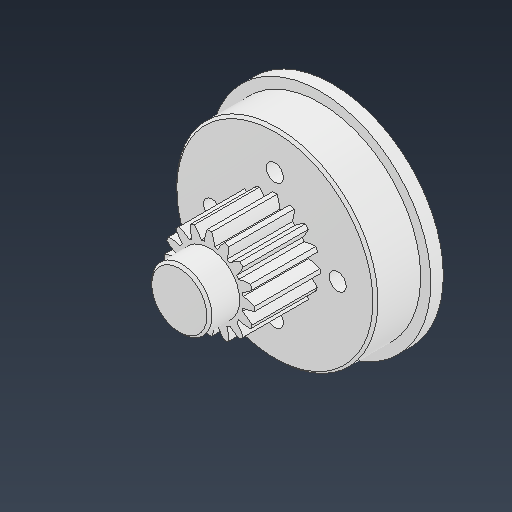
# Autodesk Inventor part: s-assy-sun_gear
Saved by Autodesk Inventor 2021 (Build 250183000, 183)
## iProperties
Created: 2021-07-12
Part Number: s-assy-sun_gear
Material: ABS プラスチック
Document SubType Name: Modeling
Designer: yuta0
Density: 1.06 g/cm^3
Appearance: 滑らか - 白
購入先: 印刷
在庫数: 0.0
Author: yuta0
Autodesk Inventor part; units mm, degrees
ref_plane "YZ Plane" through (0, 0, 0) normal (1, 0, 0) x (0, 1, 0)
ref_plane "XZ Plane" through (0, 0, 0) normal (0, 1, 0) x (-1, 0, 0)
ref_plane "XY Plane" through (0, 0, 0) normal (0, 0, 1) x (1, 0, 0)
sketch "スケッチ1" plane through (0, 0, 0) normal (1, 0, 0) x (0, 1, 0)
  line L0 (22, 0) -> (22, 2.5)
  line L1 (22, 2.5) -> (20, 2.5)
  line L2 (20, 2.5) -> (20, 11.5)
  line L3 (20, 11.5) -> (0, 11.5)
  line L4 (0, 11.5) -> (0, 0)
  line L5 (0, 0) -> (22, 0)
  dimension "d0" = 20
  dimension "d1" = 9
  dimension "d2" = 2.5
  dimension "d3" = 2
  constraints: 12 end point, 5 perpendicular, 1 vertical
  measures "d0" distance of L2.end L3.end
  measures "d1" distance of L1.end L2.end
  measures "d2" distance of L0.start L0.end
  measures "d3" distance of L0.end L1.end
revolve "回転1" add sketch "スケッチ1" angle 360 about axis through (0, 0, 11.5) along (0, 0, -1)
sketch "スケッチ2" plane through (0, 0, 11.5) normal (0, 0, 1) x (1, 0, 0)
  arc A0 (-3.8476, 8.135) -> (-3.4702, 5.7897) centre (3.494, 8.1133) ccw
  arc A1 (-3.4702, 5.7897) -> (-4.021, 5.4217) centre (0, 0) ccw
  arc A2 (-4.021, 5.4217) -> (-6.0434, 6.6678) centre (-8.8328, -0.1232) ccw
  arc A3 (-6.0434, 6.6678) -> (-6.6678, 6.0434) centre (0, 0) ccw
  arc A4 (-6.6678, 6.0434) -> (-5.4217, 4.021) centre (0.1232, 8.8328) ccw
  arc A5 (-5.4217, 4.021) -> (-5.7897, 3.4702) centre (0, 0) ccw
  arc A6 (-5.7897, 3.4702) -> (-8.135, 3.8476) centre (-8.1133, -3.494) ccw
  arc A7 (-8.135, 3.8476) -> (-8.473, 3.0317) centre (0, 0) ccw
  arc A8 (-8.473, 3.0317) -> (-6.5477, 1.6401) centre (-3.2664, 8.2076) ccw
  arc A9 (-6.5477, 1.6401) -> (-6.6769, 0.9904) centre (0, 0) ccw
  arc A10 (-6.6769, 0.9904) -> (-8.9882, 0.4416) centre (-6.1586, -6.3328) ccw
  arc A11 (-8.9882, 0.4416) -> (-8.9882, -0.4416) centre (0, 0) ccw
  arc A12 (-8.9882, -0.4416) -> (-6.6769, -0.9904) centre (-6.1586, 6.3328) ccw
  arc A13 (-6.6769, -0.9904) -> (-6.5477, -1.6401) centre (0, 0) ccw
  arc A14 (-6.5477, -1.6401) -> (-8.473, -3.0317) centre (-3.2664, -8.2076) ccw
  arc A15 (-8.473, -3.0317) -> (-8.135, -3.8476) centre (0, 0) ccw
  arc A16 (-8.135, -3.8476) -> (-5.7897, -3.4702) centre (-8.1133, 3.494) ccw
  arc A17 (-5.7897, -3.4702) -> (-5.4217, -4.021) centre (0, 0) ccw
  arc A18 (-5.4217, -4.021) -> (-6.6678, -6.0434) centre (0.1232, -8.8328) ccw
  arc A19 (-6.6678, -6.0434) -> (-6.0434, -6.6678) centre (0, 0) ccw
  arc A20 (-6.0434, -6.6678) -> (-4.021, -5.4217) centre (-8.8328, 0.1232) ccw
  arc A21 (-4.021, -5.4217) -> (-3.4702, -5.7897) centre (0, 0) ccw
  arc A22 (-3.4702, -5.7897) -> (-3.8476, -8.135) centre (3.494, -8.1133) ccw
  arc A23 (-3.8476, -8.135) -> (-3.0317, -8.473) centre (0, 0) ccw
  arc A24 (-3.0317, -8.473) -> (-1.6401, -6.5477) centre (-8.2076, -3.2664) ccw
  arc A25 (-1.6401, -6.5477) -> (-0.9904, -6.6769) centre (0, 0) ccw
  arc A26 (-0.9904, -6.6769) -> (-0.4416, -8.9882) centre (6.3328, -6.1586) ccw
  arc A27 (-0.4416, -8.9882) -> (0.4416, -8.9882) centre (0, 0) ccw
  arc A28 (0.4416, -8.9882) -> (0.9904, -6.6769) centre (-6.3328, -6.1586) ccw
  arc A29 (0.9904, -6.6769) -> (1.6401, -6.5477) centre (0, 0) ccw
  arc A30 (1.6401, -6.5477) -> (3.0317, -8.473) centre (8.2076, -3.2664) ccw
  arc A31 (3.0317, -8.473) -> (3.8476, -8.135) centre (0, 0) ccw
  arc A32 (3.8476, -8.135) -> (3.4702, -5.7897) centre (-3.494, -8.1133) ccw
  arc A33 (3.4702, -5.7897) -> (4.021, -5.4217) centre (0, 0) ccw
  arc A34 (4.021, -5.4217) -> (6.0434, -6.6678) centre (8.8328, 0.1232) ccw
  arc A35 (6.0434, -6.6678) -> (6.6678, -6.0434) centre (0, 0) ccw
  arc A36 (6.6678, -6.0434) -> (5.4217, -4.021) centre (-0.1232, -8.8328) ccw
  arc A37 (5.4217, -4.021) -> (5.7897, -3.4702) centre (0, 0) ccw
  arc A38 (5.7897, -3.4702) -> (8.135, -3.8476) centre (8.1133, 3.494) ccw
  arc A39 (8.135, -3.8476) -> (8.473, -3.0317) centre (0, 0) ccw
  arc A40 (8.473, -3.0317) -> (6.5477, -1.6401) centre (3.2664, -8.2076) ccw
  arc A41 (6.5477, -1.6401) -> (6.6769, -0.9904) centre (0, 0) ccw
  arc A42 (6.6769, -0.9904) -> (8.9882, -0.4416) centre (6.1586, 6.3328) ccw
  arc A43 (8.9882, -0.4416) -> (8.9882, 0.4416) centre (0, 0) ccw
  arc A44 (8.9882, 0.4416) -> (6.6769, 0.9904) centre (6.1586, -6.3328) ccw
  arc A45 (6.6769, 0.9904) -> (6.5477, 1.6401) centre (0, 0) ccw
  arc A46 (6.5477, 1.6401) -> (8.473, 3.0317) centre (3.2664, 8.2076) ccw
  arc A47 (8.473, 3.0317) -> (8.135, 3.8476) centre (0, 0) ccw
  arc A48 (8.135, 3.8476) -> (5.7897, 3.4702) centre (8.1133, -3.494) ccw
  arc A49 (5.7897, 3.4702) -> (5.4217, 4.021) centre (0, 0) ccw
  arc A50 (5.4217, 4.021) -> (6.6678, 6.0434) centre (-0.1232, 8.8328) ccw
  arc A51 (6.6678, 6.0434) -> (6.0434, 6.6678) centre (0, 0) ccw
  arc A52 (6.0434, 6.6678) -> (4.021, 5.4217) centre (8.8328, -0.1232) ccw
  arc A53 (4.021, 5.4217) -> (3.4702, 5.7897) centre (0, 0) ccw
  arc A54 (3.4702, 5.7897) -> (3.8476, 8.135) centre (-3.494, 8.1133) ccw
  arc A55 (3.8476, 8.135) -> (3.0317, 8.473) centre (0, 0) ccw
  arc A56 (3.0317, 8.473) -> (1.6401, 6.5477) centre (8.2076, 3.2664) ccw
  arc A57 (1.6401, 6.5477) -> (0.9904, 6.6769) centre (0, 0) ccw
  arc A58 (0.9904, 6.6769) -> (0.4416, 8.9882) centre (-6.3328, 6.1586) ccw
  arc A59 (0.4416, 8.9882) -> (-0.4416, 8.9882) centre (0, 0) ccw
  arc A60 (-0.4416, 8.9882) -> (-0.9904, 6.6769) centre (6.3328, 6.1586) ccw
  arc A61 (-0.9904, 6.6769) -> (-1.6401, 6.5477) centre (0, 0) ccw
  arc A62 (-1.6401, 6.5477) -> (-3.0317, 8.473) centre (-8.2076, 3.2664) ccw
  arc A63 (-3.0317, 8.473) -> (-3.8476, 8.135) centre (0, 0) ccw
  point P0 (0, 0)
  constraints: 128 point on circle, 64 centre point, 194 other
extrude "押し出し1" add sketch "スケッチ2" along normal blind 13
sketch "スケッチ3" plane through (0, 0, 24.5) normal (0, 0, 1) x (1, 0, 0)
  circle A0 centre (0, 0) radius 6
  dimension "d7" = 12
  constraints: 1 centre point, 1 coincident
  measures "d7" diameter of A0
extrude "押し出し2" add sketch "スケッチ3" along normal blind 6
chamfer "面取り1" distance 0.5 angle 45 2 edges at (-6, 0, 30.5) (0, -20, 11.5)
sketch "スケッチ4" plane through (0, 0, 11.5) normal (0, 0, 1) x (1, 0, 0)
  circle A0 centre (0, 0) radius 12.5
  point P0 (0, 0)
  point P1 (0, 12.5)
  point P2 (-12.5, 0)
  point P3 (0, -12.5)
  point P4 (12.5, 0)
  dimension "d13" = 25
  dimension "d16" = 360
  constraints: 1 coincident, 1 vertical alignment, 7 other
hole "穴1" at (0, 12.5, 11.5) at (-12.5, 0, 11.5) at (0, -12.5, 11.5) at (12.5, 0, 11.5) direction (0, 0, -1) diameter 3.4 end through all clearance for "Flat Head Machine Screw" size "M3" standard "Ansi Metric M Profile"
